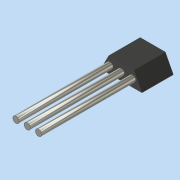
# Autodesk Inventor part: HallEffectSensor
Saved by Autodesk Inventor 2017.3 (Build 213256000, 256)
## iProperties
Created: 2018-04-12
Part Number: HallEffectSensor
Material: ABS Plastic
Document SubType Name: Modeling
Designer: Derek Wider
Density: 1.06 g/cm^3
Appearance: Smooth - Black
Author: Derek Wider
Autodesk Inventor part; units mm, degrees
ref_plane "YZ Plane" through (0, 0, 0) normal (1, 0, 0) x (0, 1, 0)
ref_plane "XZ Plane" through (0, 0, 0) normal (0, 1, 0) x (-1, 0, 0)
ref_plane "XY Plane" through (0, 0, 0) normal (0, 0, 1) x (1, 0, 0)
sketch "Sketch1" plane through (0, 0, 0) normal (0, 0, 1) x (1, 0, 0)
  line L0 (0, 0) -> (4.1656, 0)
  line L1 (4.1656, 0) -> (3.3528, 1.5748)
  line L2 (3.3528, 1.5748) -> (0.8128, 1.5748)
  line L3 (0.8128, 1.5748) -> (0, 0)
  dimension "d0" = 4.1656
  dimension "d1" = 2.54
  dimension "d2" = 1.5748
  constraints: 8 end point, 1 equal length, 1 horizontal, 1 parallel
  measures "d0" distance of L0.start L0.end
  measures "d1" distance of L1.end L2.end
  measures "d2" distance between parallel lines of L0 L2
extrude "Extrusion1" add sketch "Sketch1" along normal blind 3.175
sketch "Sketch2" plane through (0, 0, 3.175) normal (0, 0, 1) x (1, 0, 0)
  line L0 (0.8128, 1.5748) -> (0, 0) construction
  line L1 (0.4064, 0.7874) -> (3.7592, 0.7874) construction
  line L2 (4.1656, 0) -> (3.3528, 1.5748) construction
  circle A0 centre (2.0828, 0.7874) radius 0.3175
  circle A1 centre (3.2258, 0.7874) radius 0.3175
  circle A2 centre (0.9398, 0.7874) radius 0.3175
  dimension "d5" = 0.635
  dimension "d6" = 0.635
  dimension "d7" = 0.635
  dimension "d8" = 1.143
  dimension "d9" = 1.143
  constraints: 3 centre point, 3 midpoint, 2 end point, 2 point on line
  measures "d5" diameter of A0
  measures "d6" diameter of A1
  measures "d7" diameter of A2
  measures "d8" distance of A1.centre A0.centre
  measures "d9" distance of A0.centre A2.centre
extrude "Extrusion2" add sketch "Sketch2" along normal blind 9.525
equation "\"d9\" = d8"
body "Solid1"
